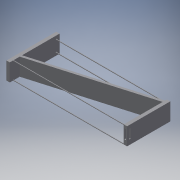
# Autodesk Inventor part: Zonnepaneel V1.0
Saved by Autodesk Inventor 2018.3 (Build 223284000, 284)
## iProperties
Created: 2020-11-12
Part Number: Zonnepaneel V1.0
Material: Generic
Document SubType Name: Modeling
Designer: daanv
Density: 1 g/cm^3
Appearance: Default
Author: daanv
Autodesk Inventor part; units mm, degrees
ref_plane "YZ Plane" through (0, 0, 0) normal (1, 0, 0) x (0, 1, 0)
ref_plane "XZ Plane" through (0, 0, 0) normal (0, 1, 0) x (-1, 0, 0)
ref_plane "XY Plane" through (0, 0, 0) normal (0, 0, 1) x (1, 0, 0)
sketch "Sketch2" plane through (0, 0, 0) normal (0, 0, 1) x (1, 0, 0)
  line L0 (0, 0) -> (100, 0)
  line L1 (100, 0) -> (100, 30)
  line L2 (100, 30) -> (0, 30)
  line L3 (0, 30) -> (0, 0)
  line L4 (100, 30) -> (103, 30)
  line L5 (103, 30) -> (103, 0)
  line L6 (103, 0) -> (100, 0)
  line L7 (100, 0) -> (100, 30)
  line L8 (0, 0) -> (-3, 0)
  line L9 (-3, 0) -> (-3, 30)
  line L10 (-3, 30) -> (0, 30)
  line L11 (0, 30) -> (0, 0)
  line L12 (0, 0) -> (103, 30)
  line L13 (103, 30) -> (102.4407, 31.9202)
  line L14 (102.4407, 31.9202) -> (-0.5593, 1.9202)
  line L15 (-0.5593, 1.9202) -> (0, 0)
  line L16 (103, 30) -> (100, 30)
  line L17 (100, 30) -> (100, 33)
  line L18 (100, 33) -> (103, 33)
  line L19 (103, 33) -> (103, 30)
  line L20 (-3, 30) -> (0, 30)
  line L21 (0, 30) -> (0, 33)
  line L22 (0, 33) -> (-3, 33)
  line L23 (-3, 33) -> (-3, 30)
  dimension "d13" = 100
  dimension "d14" = 30
  dimension "d15" = 3
  dimension "d16" = 3
  dimension "d17" = 2
  dimension "d18" = 3
  dimension "d19" = 3
  constraints: 48 end point, 12 parallel, 6 perpendicular, 5 horizontal, 1 point on line
  measures "d13" distance of L2.end L1.end
  measures "d14" distance of L1.end L0.end
  measures "d15" distance of L5.end L6.end
  measures "d16" distance of L9.end L10.end
  measures "d17" distance of L13.end L4.end
  measures "d18" distance of L16.end L17.end
  measures "d19" distance of L21.end L20.end
extrude "Extrusion2" add sketch "Sketch2" along normal blind 15.7 contours L15 L14 L3 | L3 L14 L2 L1 L12 | L8 L9 L10 L3 L14 L15 | L1 L12 L5 L6 | L1 L4 L12 | L10 L23 L22 L21 | L14 L17 L2 | L17 L14 L13 L4 | L13 L14 L17 L18 L19
sketch "Sketch4" plane through (0, 2.0831, 0) normal (1, 0, 0) x (0, 0, -1)
  line L0 (0, 30.9169) -> (-15.7, 30.9169) projected
  line L1 (-13.2, 30.9169) -> (-12.7, 30.9169)
  line L2 (-12.7, 30.9169) -> (-12.7, 30.4169)
  line L3 (-12.7, 30.4169) -> (-13.2, 30.4169)
  line L4 (-13.2, 30.4169) -> (-13.2, 30.9169)
  line L5 (-2.5, 30.9169) -> (-3, 30.9169)
  line L6 (-3, 30.9169) -> (-3, 30.4169)
  line L7 (-3, 30.4169) -> (-2.5, 30.4169)
  line L8 (-2.5, 30.4169) -> (-2.5, 30.9169)
  point P0 (0, -2.0831)
  dimension "d25" = 0.5
  dimension "d26" = 0.5
  dimension "d27" = 0.5
  constraints: 16 end point, 4 parallel, 3 point on line, 2 horizontal, 2 perpendicular
  measures "d25" distance of L2.end L3.end
  measures "d26" distance of L1.end L2.end
  measures "d27" distance of L7.end L6.end
extrude "Extrusion4" add sketch "Sketch4" along normal blind 100
sketch "Sketch5" plane through (-3, 33, 0) normal (0, 1, 0) x (1, 0, 0)
  line L0 (3, 0) -> (0, 0) projected
  line L1 (0, 0) -> (3, 0)
  line L2 (3, 0) -> (3, -15.7)
  line L3 (3, -15.7) -> (0, -15.7)
  line L4 (0, -15.7) -> (0, 0)
  constraints: 8 end point, 2 parallel, 1 horizontal, 1 perpendicular
extrude "Extrusion5" add sketch "Sketch5" along normal blind 3
sketch "Sketch6" plane through (-3, 0, 0) normal (0, -1, 0) x (1, 0, 0)
  line L0 (3, 0) -> (0, 0) projected
  line L1 (3, 0) -> (3, 15.7) projected
  line L2 (0, 15.7) -> (3, 15.7) projected
  line L3 (0, 0) -> (0, 15.7) projected
extrude "Extrusion6" add sketch "Sketch6" along normal blind 9
sketch "Sketch7" plane through (103, 33, 15.7) normal (0, 1, 0) x (1, 0, 0)
  line L0 (-0.2001, 13.2) -> (-2.7401, 13.2)
  line L1 (-2.7401, 13.2) -> (-2.7401, 2.54)
  line L2 (-2.7401, 2.54) -> (-0.2001, 2.54)
  line L3 (-0.2001, 2.54) -> (-0.2001, 13.2)
  point P0 (-103, 15.7)
  dimension "d34" = 2.54
  dimension "d35" = 10.66
  constraints: 8 end point, 2 parallel, 1 horizontal, 1 perpendicular
  measures "d34" distance of L2.end L1.end
  measures "d35" distance of L1.end L0.end
extrude "Extrusion7" cut sketch "Sketch7" against normal blind 12
sketch "Sketch8" plane through (100, 29.1262, 0) normal (-1, 0, 0) x (0, 0, 1)
  line L0 (13.16, 3.8738) -> (13.16, -8.1262) projected
  line L1 (2.5, 3.8738) -> (2.5, -8.1262) projected
  line L2 (13.16, -8.1262) -> (2.5, -8.1262)
  line L3 (2.5, -8.1262) -> (2.5, -4.1262)
  line L4 (2.5, -4.1262) -> (13.16, -4.1262)
  line L5 (13.16, -4.1262) -> (13.16, -8.1262)
  point P0 (0, -29.1262)
  dimension "d38" = 4
  constraints: 8 end point, 2 parallel, 1 horizontal, 1 perpendicular, 1 point on line
  measures "d38" distance of L2.end L3.end
extrude "Extrusion8" cut sketch "Sketch8" against normal blind 1
sketch "Sketch9" plane through (0, 2.0831, 15.7) normal (-0.2796, 0.9601, 0) x (0.9601, 0.2796, 0)
  line L0 (0, 0) -> (0, 15.7) projected
  line L1 (104.1553, 15.7) -> (104.1553, 0) projected
  line L2 (104.1553, 15.7) -> (0, 15.7)
  line L3 (0, 15.7) -> (0, 15.6)
  line L4 (0, 15.6) -> (104.1553, 15.6)
  line L5 (104.1553, 15.6) -> (104.1553, 15.7)
  line L6 (104.1553, 15.3) -> (0, 15.3)
  line L7 (0, 15.3) -> (0, 15.2)
  line L8 (0, 15.2) -> (104.1553, 15.2)
  line L9 (104.1553, 15.2) -> (104.1553, 15.3)
  line L10 (104.1553, 14.9) -> (0, 14.9)
  line L11 (0, 14.9) -> (0, 14.8)
  line L12 (0, 14.8) -> (104.1553, 14.8)
  line L13 (104.1553, 14.8) -> (104.1553, 14.9)
  line L14 (104.1553, 14.5) -> (0, 14.5)
  line L15 (0, 14.5) -> (0, 14.4)
  line L16 (0, 14.4) -> (104.1553, 14.4)
  line L17 (104.1553, 14.4) -> (104.1553, 14.5)
  line L18 (104.1553, 14.1) -> (0, 14.1)
  line L19 (0, 14.1) -> (0, 14)
  line L20 (0, 14) -> (104.1553, 14)
  line L21 (104.1553, 14) -> (104.1553, 14.1)
  line L22 (104.1553, 13.7) -> (0, 13.7)
  line L23 (0, 13.7) -> (0, 13.6)
  line L24 (0, 13.6) -> (104.1553, 13.6)
  line L25 (104.1553, 13.6) -> (104.1553, 13.7)
  line L26 (104.1553, 13.3) -> (0, 13.3)
  line L27 (0, 13.3) -> (0, 13.2)
  line L28 (0, 13.2) -> (104.1553, 13.2)
  line L29 (104.1553, 13.2) -> (104.1553, 13.3)
  line L30 (104.1553, 12.9) -> (0, 12.9)
  line L31 (0, 12.9) -> (0, 12.8)
  line L32 (0, 12.8) -> (104.1553, 12.8)
  line L33 (104.1553, 12.8) -> (104.1553, 12.9)
  line L34 (104.1553, 12.5) -> (0, 12.5)
  line L35 (0, 12.5) -> (0, 12.4)
  line L36 (0, 12.4) -> (104.1553, 12.4)
  line L37 (104.1553, 12.4) -> (104.1553, 12.5)
  line L38 (104.1553, 12.1) -> (0, 12.1)
  line L39 (0, 12.1) -> (0, 12)
  line L40 (0, 12) -> (104.1553, 12)
  line L41 (104.1553, 12) -> (104.1553, 12.1)
  line L42 (104.1553, 11.7) -> (0, 11.7)
  line L43 (0, 11.7) -> (0, 11.6)
  line L44 (0, 11.6) -> (104.1553, 11.6)
  line L45 (104.1553, 11.6) -> (104.1553, 11.7)
  line L46 (104.1553, 11.3) -> (0, 11.3)
  line L47 (0, 11.3) -> (0, 11.2)
  line L48 (0, 11.2) -> (104.1553, 11.2)
  line L49 (104.1553, 11.2) -> (104.1553, 11.3)
  line L50 (104.1553, 10.9) -> (0, 10.9)
  line L51 (0, 10.9) -> (0, 10.8)
  line L52 (0, 10.8) -> (104.1553, 10.8)
  line L53 (104.1553, 10.8) -> (104.1553, 10.9)
  line L54 (104.1553, 10.5) -> (0, 10.5)
  line L55 (0, 10.5) -> (0, 10.4)
  line L56 (0, 10.4) -> (104.1553, 10.4)
  line L57 (104.1553, 10.4) -> (104.1553, 10.5)
  line L58 (104.1553, 10.1) -> (0, 10.1)
  line L59 (0, 10.1) -> (0, 10)
  line L60 (0, 10) -> (104.1553, 10)
  line L61 (104.1553, 10) -> (104.1553, 10.1)
  line L62 (104.1553, 9.7) -> (0, 9.7)
  line L63 (0, 9.7) -> (0, 9.6)
  line L64 (0, 9.6) -> (104.1553, 9.6)
  line L65 (104.1553, 9.6) -> (104.1553, 9.7)
  line L66 (104.1553, 9.3) -> (0, 9.3)
  line L67 (0, 9.3) -> (0, 9.2)
  line L68 (0, 9.2) -> (104.1553, 9.2)
  line L69 (104.1553, 9.2) -> (104.1553, 9.3)
  line L70 (104.1553, 8.9) -> (0, 8.9)
  line L71 (0, 8.9) -> (0, 8.8)
  line L72 (0, 8.8) -> (104.1553, 8.8)
  line L73 (104.1553, 8.8) -> (104.1553, 8.9)
  line L74 (104.1553, 8.5) -> (0, 8.5)
  line L75 (0, 8.5) -> (0, 8.4)
  line L76 (0, 8.4) -> (104.1553, 8.4)
  line L77 (104.1553, 8.4) -> (104.1553, 8.5)
  line L78 (104.1553, 8.1) -> (0, 8.1)
  line L79 (0, 8.1) -> (0, 8)
  line L80 (0, 8) -> (104.1553, 8)
  line L81 (104.1553, 8) -> (104.1553, 8.1)
  line L82 (104.1553, 7.7) -> (0, 7.7)
  line L83 (0, 7.7) -> (0, 7.6)
  line L84 (0, 7.6) -> (104.1553, 7.6)
  line L85 (104.1553, 7.6) -> (104.1553, 7.7)
  line L86 (104.1553, 7.3) -> (0, 7.3)
  line L87 (0, 7.3) -> (0, 7.2)
  line L88 (0, 7.2) -> (104.1553, 7.2)
  line L89 (104.1553, 7.2) -> (104.1553, 7.3)
  line L90 (104.1553, 6.9) -> (0, 6.9)
  line L91 (0, 6.9) -> (0, 6.8)
  line L92 (0, 6.8) -> (104.1553, 6.8)
  line L93 (104.1553, 6.8) -> (104.1553, 6.9)
  line L94 (104.1553, 6.5) -> (0, 6.5)
  line L95 (0, 6.5) -> (0, 6.4)
  line L96 (0, 6.4) -> (104.1553, 6.4)
  line L97 (104.1553, 6.4) -> (104.1553, 6.5)
  line L98 (104.1553, 6.1) -> (0, 6.1)
  line L99 (0, 6.1) -> (0, 6)
  line L100 (0, 6) -> (104.1553, 6)
  line L101 (104.1553, 6) -> (104.1553, 6.1)
  line L102 (104.1553, 5.7) -> (0, 5.7)
  line L103 (0, 5.7) -> (0, 5.6)
  line L104 (0, 5.6) -> (104.1553, 5.6)
  line L105 (104.1553, 5.6) -> (104.1553, 5.7)
  line L106 (104.1553, 5.3) -> (0, 5.3)
  line L107 (0, 5.3) -> (0, 5.2)
  line L108 (0, 5.2) -> (104.1553, 5.2)
  line L109 (104.1553, 5.2) -> (104.1553, 5.3)
  line L110 (104.1553, 4.9) -> (0, 4.9)
  line L111 (0, 4.9) -> (0, 4.8)
  line L112 (0, 4.8) -> (104.1553, 4.8)
  line L113 (104.1553, 4.8) -> (104.1553, 4.9)
  line L114 (104.1553, 4.5) -> (0, 4.5)
  line L115 (0, 4.5) -> (0, 4.4)
  line L116 (0, 4.4) -> (104.1553, 4.4)
  line L117 (104.1553, 4.4) -> (104.1553, 4.5)
  line L118 (104.1553, 4.1) -> (0, 4.1)
  line L119 (0, 4.1) -> (0, 4)
  line L120 (0, 4) -> (104.1553, 4)
  line L121 (104.1553, 4) -> (104.1553, 4.1)
  line L122 (104.1553, 3.7) -> (0, 3.7)
  line L123 (0, 3.7) -> (0, 3.6)
  line L124 (0, 3.6) -> (104.1553, 3.6)
  line L125 (104.1553, 3.6) -> (104.1553, 3.7)
  line L126 (104.1553, 3.3) -> (0, 3.3)
  line L127 (0, 3.3) -> (0, 3.2)
  line L128 (0, 3.2) -> (104.1553, 3.2)
  line L129 (104.1553, 3.2) -> (104.1553, 3.3)
  line L130 (104.1553, 2.9) -> (0, 2.9)
  line L131 (0, 2.9) -> (0, 2.8)
  line L132 (0, 2.8) -> (104.1553, 2.8)
  line L133 (104.1553, 2.8) -> (104.1553, 2.9)
  line L134 (104.1553, 2.5) -> (0, 2.5)
  line L135 (0, 2.5) -> (0, 2.4)
  line L136 (0, 2.4) -> (104.1553, 2.4)
  line L137 (104.1553, 2.4) -> (104.1553, 2.5)
  line L138 (104.1553, 2.1) -> (0, 2.1)
  line L139 (0, 2.1) -> (0, 2)
  line L140 (0, 2) -> (104.1553, 2)
  line L141 (104.1553, 2) -> (104.1553, 2.1)
  line L142 (104.1553, 1.7) -> (0, 1.7)
  line L143 (0, 1.7) -> (0, 1.6)
  line L144 (0, 1.6) -> (104.1553, 1.6)
  line L145 (104.1553, 1.6) -> (104.1553, 1.7)
  line L146 (104.1553, 1.3) -> (0, 1.3)
  line L147 (0, 1.3) -> (0, 1.2)
  line L148 (0, 1.2) -> (104.1553, 1.2)
  line L149 (104.1553, 1.2) -> (104.1553, 1.3)
  line L150 (104.1553, 0.9) -> (0, 0.9)
  line L151 (0, 0.9) -> (0, 0.8)
  line L152 (0, 0.8) -> (104.1553, 0.8)
  line L153 (104.1553, 0.8) -> (104.1553, 0.9)
  line L154 (104.1553, 0.5) -> (0, 0.5)
  line L155 (0, 0.5) -> (0, 0.4)
  line L156 (0, 0.4) -> (104.1553, 0.4)
  line L157 (104.1553, 0.4) -> (104.1553, 0.5)
  line L158 (104.1553, 0.1) -> (0, 0.1)
  line L159 (0, 0.1) -> (0, 0)
  line L160 (0, 0) -> (104.1553, 0)
  line L161 (104.1553, 0) -> (104.1553, 0.1)
  point P0 (-0.5825, 15.7)
  dimension "d41" = 0.1
  dimension "d44" = 0.4
  constraints: 320 end point, 2 parallel, 1 horizontal, 1 perpendicular, 1 point on line, 1 vertical, 312 other
  measures "d41" distance of L3.end L2.end
  measures "d44" distance of L3.end L7.end
extrude "Extrusion9" add sketch "Sketch9" along normal blind 0.05 contours L0 L158 L1 L160 | L0 L154 L1 L156 | L0 L150 L1 L152 | L0 L146 L1 L148 | L0 L142 L1 L144 | L0 L138 L1 L140 | L0 L134 L1 L136 | L0 L130 L1 L132 | L0 L126 L1 L128 | L0 L122 L1 L124 | L0 L118 L1 L120 | L0 L114 L1 L116 | L0 L110 L1 L112 | L0 L106 L1 L108 | L0 L102 L1 L104 | L0 L98 L1 L100 | L0 L94 L1 L96 | L0 L90 L1 L92 | L0 L86 L1 L88 | L0 L82 L1 L84 | L0 L78 L1 L80 | L0 L74 L1 L76 | L0 L70 L1 L72 | L0 L66 L1 L68 | L0 L62 L1 L64 | L0 L58 L1 L60 | L0 L54 L1 L56 | L0 L50 L1 L52 | L0 L46 L1 L48 | L0 L42 L1 L44 | L0 L38 L1 L40 | L0 L34 L1 L36 | L0 L30 L1 L32 | L0 L26 L1 L28 | L0 L22 L1 L24 | L0 L18 L1 L20 | L0 L14 L1 L16 | L0 L10 L1 L12 | L0 L6 L1 L8 | L0 L2 L1 L4
sketch "Sketch11" plane through (100, 0, 0) normal (0, -1, 0) x (1, 0, 0)
  line L0 (3, 0) -> (0, 0) projected
  line L1 (3, 0) -> (3, 15.7) projected
  line L2 (0, 15.7) -> (3, 15.7) projected
  line L3 (0, 0) -> (0, 15.7) projected
  point P0 (-100, 0)
extrude "Extrusion10" add sketch "Sketch11" along normal blind 6
sketch "Sketch12" plane through (0, -9, 15.7) normal (1, 0, 0) x (0, 0, -1)
  line L0 (0, 9) -> (0, 0) projected
  line L1 (15.7, 9) -> (15.7, 0) projected
  line L2 (0, 3.5) -> (0.5, 3.5)
  line L3 (0.5, 3.5) -> (0.5, 3)
  line L4 (0.5, 3) -> (0, 3)
  line L5 (0, 3) -> (0, 3.5)
  line L6 (15.7, 3.5) -> (15.2, 3.5)
  line L7 (15.2, 3.5) -> (15.2, 3)
  line L8 (15.2, 3) -> (15.7, 3)
  line L9 (15.7, 3) -> (15.7, 3.5)
  line L10 (15.7, 0) -> (0, 0) projected
  dimension "d53" = 0.5
  dimension "d54" = 0.5
  dimension "d55" = 0.5
  dimension "d56" = 0.5
  dimension "d59" = 3
  constraints: 16 end point, 4 parallel, 3 point on line, 2 horizontal, 2 perpendicular
  measures "d53" distance of L3.end L4.end
  measures "d54" distance of L2.end L3.end
  measures "d55" distance of L8.end L7.end
  measures "d56" distance of L7.end L6.end
  measures "d59" distance between parallel lines of L10 L4
extrude "Extrusion11" add sketch "Sketch12" along normal blind 100
sketch "Sketch16" plane through (100, -6, 0) normal (0, -1, 0) x (1, 0, 0)
  line L0 (-100, 0) -> (3, 0) projected
  line L1 (3, 15.7) -> (-100, 15.7) projected
  line L2 (0.5142, 12.8501) -> (1.5142, 12.8501)
  line L3 (1.5142, 12.8501) -> (1.5142, 2.8501)
  line L4 (1.5142, 2.8501) -> (0.5142, 2.8501)
  line L5 (0.5142, 2.8501) -> (0.5142, 12.8501)
  dimension "d73" = 1
  dimension "d74" = 10
  dimension "d75" = 2.8501
  dimension "d76" = 2.8499
  constraints: 8 end point, 2 parallel, 1 horizontal, 1 perpendicular
  measures "d73" distance of L3.end L4.end
  measures "d74" distance of L2.end L3.end
  measures "d75" distance between parallel lines of L0 L4
  measures "d76" distance between parallel lines of L1 L2
extrude "Extrusion15" cut sketch "Sketch16" against normal blind 4.7
sketch "Sketch17" plane through (100, -6, 0) normal (0, -1, 0) x (1, 0, 0)
  line L0 (0.489, 13.8501) -> (0.989, 14.7161)
  line L1 (0.489, 13.8501) -> (1.489, 13.8501) construction
  line L2 (0.989, 14.7161) -> (1.5142, 13.8501)
  line L3 (1.5142, 13.8501) -> (0.489, 13.8501)
  line L4 (0.5142, 12.8501) -> (1.5142, 12.8501) projected
  dimension "d79" = 1
  dimension "d80" = 60
  dimension "d89" = 1
  constraints: 8 end point, 2 horizontal, 1 equal length
  measures "d79" distance of L0.start L0.end
  measures "d80" angle of L1 L0
  measures "d89" distance between parallel lines of L4 L1
extrude "Extrusion16" add sketch "Sketch17" along normal blind 3
sketch "Sketch18" plane through (100, -6, 0) normal (0, -1, 0) x (1, 0, 0)
  line L0 (1.5142, 2.8501) -> (0.5142, 2.8501) projected
  line L1 (0.5142, 1.8501) -> (1.5142, 1.8501)
  line L2 (1.5142, 1.8501) -> (1.5142, 0.8501)
  line L3 (1.5142, 0.8501) -> (0.5142, 0.8501)
  line L4 (0.5142, 0.8501) -> (0.5142, 1.8501)
  dimension "d83" = 1
  dimension "d84" = 1
  dimension "d85" = 1
  constraints: 8 end point, 2 parallel, 1 horizontal, 1 perpendicular
  measures "d83" distance of L2.end L3.end
  measures "d84" distance of L1.end L2.end
  measures "d85" distance between parallel lines of L0 L1
extrude "Extrusion17" add sketch "Sketch18" along normal blind 3
chamfer "Chamfer1" distance 0.29 angle 45 3 edges at (101.2516, -9, 14.2831) (100.739, -9, 14.2831) (101.0016, -9, 13.8501)
chamfer "Chamfer2" distance 0.499 angle 45 4 edges at (100.5142, -9, 1.3501) (101.0142, -9, 1.8501) (101.5142, -9, 1.3501) (101.0142, -9, 0.8501)
chamfer "Chamfer3" distance 0.499 angle 45 4 edges at (101.0142, -8.501, 1.8501) (101.5142, -8.501, 1.3501) (101.0142, -8.501, 0.8501) (100.5142, -8.501, 1.3501)
chamfer "Chamfer4" distance 0.29 angle 45 3 edges at (101.2516, -8.71, 14.2831) (100.739, -8.71, 14.2831) (101.0016, -8.71, 13.8501)
body "Solid2"
